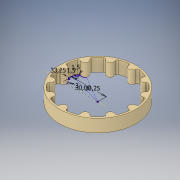
# Autodesk Inventor part: Enclosure
Saved by Autodesk Inventor 2018.3 (Build 223284000, 284)
## iProperties
Created: 2018-07-20
Part Number: Enclosure
Material: Generisch
Document SubType Name: Modeling
Designer: JochenAlt
Density: 1 g/cm^3
Appearance: Weizen
Author: JochenAlt
Autodesk Inventor part; units mm, degrees
ref_plane "YZ Plane" through (0, 0, 0) normal (1, 0, 0) x (0, 1, 0)
ref_plane "XZ Plane" through (0, 0, 0) normal (0, 1, 0) x (-1, 0, 0)
ref_plane "XY Plane" through (0, 0, 0) normal (0, 0, 1) x (1, 0, 0)
sketch "Skizze1" plane through (0, 0, 0) normal (0, 0, 1) x (1, 0, 0)
  line L0 (-46.7955, 0) -> (7.7993, 0) construction
  arc A0 (-28.7953, 16.625) -> (-33.25, 0) centre (0, 0) ccw
  arc A1 (-27.25, 0) -> (-29.9525, 2.9852) centre (-30.25, 0) ccw
  line L1 (0, 0) -> (-38.9963, 22.5145) construction
  line L2 (-30.25, 0) -> (0, 0) construction
  arc A2 (-27.4322, 12.391) -> (-23.5992, 13.625) centre (-26.1973, 15.125) ccw
  arc A3 (-29.75, 5.4772) -> (-30.25, 0) centre (0, 0) ccw construction
  arc A4 (-26.1973, 15.125) -> (-29.75, 5.4772) centre (0, 0) ccw construction
  line L3 (-37.9513, 10.169) -> (0, 0) construction
  line L4 (-23.5992, 13.625) -> (-28.7953, 16.625)
  line L5 (-27.25, 0) -> (-33.25, 0)
  line L6 (-27.4322, 12.391) -> (-27.5342, 12.437)
  line L7 (-29.9525, 2.9852) -> (-30.0638, 2.9963)
  arc A5 (-29.5476, 11.619) -> (-31.3985, 4.7115) centre (0, 0) ccw
  arc A6 (-27.5342, 12.437) -> (-29.5476, 11.619) centre (-28.1517, 11.07) ccw
  arc A7 (-31.3985, 4.7115) -> (-30.0638, 2.9963) centre (-29.9151, 4.4889) ccw
  point P0 (-29.2193, 7.8293)
  point P1 (-28.9351, 13.0698)
  point P2 (-31.5935, 3.1488)
  dimension "d5" = 3
  dimension "d14" = 30.25
  dimension "d28" = 30
  dimension "d38" = 1.5
  dimension "d39" = 1.5
  dimension "d40" = 33.25
  constraints: 20 point on circle, 14 end point, 9 point on line, 8 centre point, 6 tangent, 3 coincident, 2 collinear, 2 equal radius, 1 other
  measures "d5" radius of A1
  measures "d14" distance of L1.start L2.start
  measures "d28" angle of L1 L0
  measures "d38" radius of A6
  measures "d39" radial gap between concentric circles of A5 A4
  measures "d40" radius of A0
extrude "Extrusion1" add sketch "Skizze1" along normal blind 11
pattern_circular "Runde Anordnung1" count 12 over 360 about axis through (0, 0, 0) along (0, 0, 1) of "Extrusion1"
